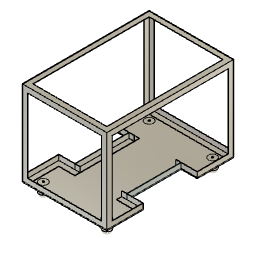
sentry_frame v40 (Autodesk Fusion 360 design; units mm, degrees)
Autodesk Fusion 360 part; units mm, degrees
sketch "1-inch Frame Profile" plane through (0, 0, 0) normal (0, 1, 0) x (1, 0, 0)
  line L0 (-200, -27.4) -> (-200, -2)
  line L1 (-200, -2) -> (-174.6, -2)
  line L2 (-174.6, -2) -> (-174.6, -27.4)
  line L3 (-174.6, -27.4) -> (-200, -27.4)
  line L4 (-174.6, -27.4) -> (-198, -27.4)
  line L5 (-198, -27.4) -> (-198, -4)
  line L6 (-198, -4) -> (-174.6, -4)
  line L7 (-174.6, -4) -> (-174.6, -27.4)
  dimension "d5" = 25.4
  dimension "d6" = 25.4
  dimension "d7" = 23.4
  dimension "d8" = 23.4
  constraint perpendicular L0 L1
  constraint parallel L0 L2
  constraint parallel L1 L3
  constraint vertical L0
  constraint horizontal L4
  constraint vertical L5
  constraint horizontal L6
  constraint vertical L7
  measures "d5" distance of L0.start L2.end
  measures "d6" distance of L1 L3
  measures "d7" distance of L2.end L4.end
  measures "d8" distance of L2.end L6.end
extrude "Extrude3" add sketch "1-inch Frame Profile" along normal blind 600 contours L0 L1 L2 L3 L5 L6 makes body 1
move_body "Move1" bodies 1 to x (1, 0, 0) y (0, 1, 0) z (0, 0, 1) at (0, -300, 0)
copy_body "CopyPasteBodies1" bodies 1 makes body 2
move_body "Move2" bodies 2 to x (-1, 0, 0) y (0, -1, 0) z (0, 0, 1) at (-400, -600, 0)
move_body "Move3" bodies 2 to x (1, 0, 0) y (0, 1, 0) z (0, 0, 1) at (400, 600, 0)
extrude "Extrude5" add sketch "1-inch Frame Profile" along normal blind 400 separate body contours L0 L1 L2 L3 L5 L6 makes body 3
move_body "Move8" bodies 3 to x (0, 1, 0) y (-1, 0, 0) z (0, 0, 1) at (-200, 200, 0)
move_body "Move9" bodies 3 to x (1, 0, 0) y (0, 1, 0) z (0, 0, 1) at (400, -300, 0)
copy_body "CopyPasteBodies4" bodies 3 makes body 4
move_body "Move10" bodies 4 to x (-1, 0, 0) y (0, -1, 0) z (0, 0, 1) at (0, 0, 0)
move_body "Move11" bodies 1 3 4 2 to x (-1, 0, 0) y (0, 1, 0) z (0, 0, -1) at (0, 0, 4)
move_body "Move12" bodies 1 3 4 2 to x (1, 0, 0) y (0, 1, 0) z (0, 0, 1) at (0, 0, 400)
copy_body "CopyPasteBodies5" bodies 3 4 makes body 5 makes body 6
move_body "Move13" bodies 5 6 to x (-1, 0, 0) y (0, 1, 0) z (0, 0, -1) at (0, 0, 778.6)
move_body "Move14" bodies 5 6 to x (1, 0, 0) y (0, 1, 0) z (0, 0, 1) at (0, 0, -375)
extrude "Extrude6" add sketch "1-inch Frame Profile" along normal blind 173 separate body contours L0 L1 L2 L3 L5 L6 makes body 7
move_body "Move15" bodies 7 to x (1, 0, 0) y (0, 1, 0) z (0, 0, 1) at (0, -300, 0)
copy_body "CopyPasteBodies6" bodies 7 makes body 8
move_body "Move16" bodies 8 to x (1, 0, 0) y (0, 1, 0) z (0, 0, 1) at (0, 427, 0)
copy_body "CopyPasteBodies7" bodies 7 8 makes body 9 makes body 10
move_body "Move17" bodies 9 10 to x (-1, 0, 0) y (0, -1, 0) z (0, 0, 1) at (0, 0, 0)
extrude "Extrude7" add sketch "1-inch Frame Profile" along normal blind 101.6 separate body contours L0 L1 L2 L3 L5 L6 makes body 11
move_body "Move18" bodies 11 to x (0, -1, 0) y (1, 0, 0) z (0, 0, 1) at (-200, -327, 0)
copy_body "CopyPasteBodies8" bodies 11 makes body 12
move_body "Move19" bodies 12 to x (-1, 0, 0) y (0, -1, 0) z (0, 0, 1) at (-300, 5.2, 0)
move_body "Move20" bodies 12 to x (1, 0, 0) y (0, 1, 0) z (0, 0, 1) at (1.6, -5.2, 0)
extrude "Extrude8" add sketch "1-inch Frame Profile" along normal blind 254 separate body contours L0 L1 L2 L3 L5 L6 makes body 13
move_body "Move21" bodies 13 to x (1, 0, 0) y (0, 1, 0) z (0, 0, 1) at (76.2, -127, 0)
combine "Combine1" operation add target body 11 tool bodies 13 12
copy_body "CopyPasteBodies9" bodies 11 makes body 14
move_body "Move22" bodies 14 to x (-1, 0, 0) y (0, -1, 0) z (0, 0, 1) at (0, 0, 0)
combine "Combine2" operation add target body 14 tool bodies 9 11 10 7 5 6 8
combine "Combine3" operation add target body 1 tool bodies 4 3 2
extrude "Extrude9" add sketch "1-inch Frame Profile" along normal blind 400 separate body contours L0 L1 L2 L3 L5 L6 makes body 15
move_body "Move23" bodies 15 to x (1, 0, 0) y (0, 0, 1) z (0, -1, 0) at (0, 302, 2)
copy_body "CopyPasteBodies10" bodies 15 makes body 16
move_body "Move24" bodies 16 to x (0, 1, 0) y (-1, 0, 0) z (0, 0, 1) at (99.6, -100, 0)
move_body "Move25" bodies 16 to x (1, 0, 0) y (0, 1, 0) z (0, 0, 1) at (0.4, 0, 0)
copy_body "CopyPasteBodies11" bodies 15 16 makes body 17 makes body 18
move_body "Move26" bodies 17 18 to x (-1, 0, 0) y (0, -1, 0) z (0, 0, 1) at (0, -0.8, 0)
move_body "Move27" bodies 17 18 to x (1, 0, 0) y (0, 1, 0) z (0, 0, 1) at (0, 0.8, 0)
sketch "Sketch7" plane through (0, 0, 0) normal (0, 0, 1) x (1, 0, 0)
  line L0 (-200, 300) -> (200, 300)
  line L1 (200, 300) -> (200, -300)
  line L2 (200, -300) -> (-200, -300)
  line L3 (-200, -300) -> (-200, 300)
  line L4 (123.8, -127) -> (200, -127)
  line L5 (200, -127) -> (200, 127.0447)
  line L6 (200, 127.0447) -> (123.8, 127.0447)
  line L7 (123.8, 127.0447) -> (123.8, -127)
  line L8 (-123.8, -127) -> (-200, -127)
  line L9 (-200, -127) -> (-200, 126.9617)
  line L10 (-200, 126.9617) -> (-123.8, 126.9617)
  line L11 (-123.8, 126.9617) -> (-123.8, -127)
  constraint horizontal L0
  constraint vertical L1
  constraint horizontal L2
  constraint vertical L3
  constraint perpendicular L4 L5
  constraint parallel L4 L6
  constraint parallel L5 L7
  constraint coincident L1 L4.end
  constraint perpendicular L1 L4
  constraint perpendicular L8 L9
  constraint parallel L8 L10
  constraint parallel L9 L11
  constraint coincident L3 L8.end
  constraint perpendicular L3 L8
extrude "Extrude10" add sketch "Sketch7" along normal blind 2 separate body contours L0 L1 L2 L3 L4 L6 L7 L8 L10 L11 makes body 19
sketch "Sketch9" plane through (0, 0, 2) normal (0, 0, 1) x (-1, 0, 0)
  line L0 (200, -126.9617) -> (123.8, -126.9617)
  line L1 (123.8, -126.9617) -> (123.8, 127)
  line L2 (123.8, 127) -> (200, 127)
  line L3 (200, 127) -> (200, 300)
  line L4 (200, 300) -> (-200, 300)
  line L5 (-200, 300) -> (-200, 127)
  line L6 (-200, 127) -> (-123.8, 127)
  line L7 (-123.8, 127) -> (-123.8, -127.0447)
  line L8 (-123.8, -127.0447) -> (-200, -127.0447)
  line L9 (-200, -127.0447) -> (-200, -300)
  line L10 (-200, -300) -> (200, -300)
  line L11 (200, -300) -> (200, -126.9617)
  circle A0 centre (150, 250) radius 4.25
  circle A1 centre (-150, 250) radius 4.25
  circle A2 centre (150, -250) radius 4.25
  circle A3 centre (-150, -250) radius 4.25
  dimension "d30" = 8.5
  dimension "d31" = 8.5
  dimension "d32" = 8.5
  dimension "d33" = 8.5
  measures "d30" diameter of A0
  measures "d31" diameter of A1
  measures "d32" diameter of A2
  measures "d33" diameter of A3
extrude "Extrude12" cut sketch "Sketch9" against normal blind 10 contours A0 | A1 | A2 | A3 bodies 19
combine "Combine4" operation add target body 1 tool bodies 18 17 14 15 16
copy_body "Body->Comp4" bodies 1 removing the originals makes body 20 in component "base_link"
sketch "Sketch14" plane through (123.8, 0, 0) normal (1, 0, 0) x (0, 1, 0)
  line L0 (127, 62) -> (127, 87.4)
  line L1 (127, 87.4) -> (-127, 87.4)
  line L2 (-127, 87.4) -> (-127, 62)
  line L3 (-127, 62) -> (127, 62)
sketch "Sketch17" plane through (-123.8, 0, 0) normal (-1, 0, 0) x (0, -1, 0)
  line L0 (127, 62) -> (127, 87.4)
  line L1 (127, 87.4) -> (-127, 87.4)
  line L2 (-127, 87.4) -> (-127, 62)
  line L3 (-127, 62) -> (127, 62)
sketch "Sketch18" plane through (0, 0, 0) normal (1, 0, 0) x (0, 1, 0)
  circle A0 centre (0, 73) radius 4.4721
copy_body "CutPasteBodies4" bodies 19 body 19 seen with x (1, 0, 0) y (0, 1, 0) z (0, 0, 1) at (0, 0, -60) removing the originals makes body 21 in component "base_link"
move_body "Move3'" bodies 21 to x (1, 0, 0) y (0, 1, 0) z (0, 0, 1) at (0, 0, 60) in component "base_link"
combine "Combine2'" operation add target body 21 tool bodies 20 in component "base_link"
sketch "Sketch30" plane through (0, 0, 60) normal (0, 0, -1) x (1, 0, 0)
  circle A0 centre (150, 250) radius 4.25
  circle A1 centre (150, -250) radius 4.25
  circle A2 centre (-150, 250) radius 4.25
  circle A3 centre (-150, -250) radius 4.25
  line L0 (-123.8, -126.9617) -> (-200, -126.9617)
  line L1 (-200, -126.9617) -> (-200, -300)
  line L2 (-200, -300) -> (200, -300)
  line L3 (200, -300) -> (200, -127.0447)
  line L4 (200, -127.0447) -> (123.8, -127.0447)
  line L5 (123.8, -127.0447) -> (123.8, 127)
  line L6 (123.8, 127) -> (200, 127)
  line L7 (200, 127) -> (200, 300)
  line L8 (200, 300) -> (-200, 300)
  line L9 (-200, 300) -> (-200, 127)
  line L10 (-200, 127) -> (-123.8, 127)
  line L11 (-123.8, 127) -> (-123.8, -126.9617)
  circle A4 centre (-150, 250) radius 20
  dimension "d284" = 40
  constraint concentric A2 A4
  measures "d284" diameter of A4
extrude "Extrude1" add sketch "Sketch30" along normal blind 60 contours A2 | A4 sketch seen with x (1, 0, 0) y (0, 1, 0) z (0, 0, 1) at (0, 0, -60) bodies 21 in component "base_link"
fillet "Fillet1" radius 20 1 edges at (-168.6465, -242.7677, -60) on bodies 21 in component "base_link"
sketch "Sketch31" plane through (0, 0, 60) normal (0, 0, -1) x (1, 0, 0)
  circle A0 centre (-150, 250) radius 20
  circle A1 centre (150, 250) radius 4.25
  circle A2 centre (150, -250) radius 4.25
  circle A3 centre (-150, -250) radius 4.25
  line L0 (-123.8, -126.9617) -> (-200, -126.9617)
  line L1 (-200, -126.9617) -> (-200, -300)
  line L2 (-200, -300) -> (200, -300)
  line L3 (200, -300) -> (200, -127.0447)
  line L4 (200, -127.0447) -> (123.8, -127.0447)
  line L5 (123.8, -127.0447) -> (123.8, 127)
  line L6 (123.8, 127) -> (200, 127)
  line L7 (200, 127) -> (200, 300)
  line L8 (200, 300) -> (-200, 300)
  line L9 (-200, 300) -> (-200, 127)
  line L10 (-200, 127) -> (-123.8, 127)
  line L11 (-123.8, 127) -> (-123.8, -126.9617)
  circle A4 centre (150, 250) radius 20
  dimension "d289" = 40
  constraint concentric A1 A4
  measures "d289" diameter of A4
extrude "Extrude2" add sketch "Sketch31" along normal blind 60 contours A1 | A4 sketch seen with x (1, 0, 0) y (0, 1, 0) z (0, 0, 1) at (0, 0, -60) bodies 21 in component "base_link"
fillet "Fillet2" radius 20 1 faces at (156.1685, -243.352, -60) on bodies 21 in component "base_link"
sketch "Sketch32" plane through (0, 0, 60) normal (0, 0, -1) x (1, 0, 0)
  circle A0 centre (150, 250) radius 20
  circle A1 centre (-150, 250) radius 20
  circle A2 centre (150, -250) radius 4.25
  circle A3 centre (-150, -250) radius 4.25
  line L0 (-123.8, -126.9617) -> (-200, -126.9617)
  line L1 (-200, -126.9617) -> (-200, -300)
  line L2 (-200, -300) -> (200, -300)
  line L3 (200, -300) -> (200, -127.0447)
  line L4 (200, -127.0447) -> (123.8, -127.0447)
  line L5 (123.8, -127.0447) -> (123.8, 127)
  line L6 (123.8, 127) -> (200, 127)
  line L7 (200, 127) -> (200, 300)
  line L8 (200, 300) -> (-200, 300)
  line L9 (-200, 300) -> (-200, 127)
  line L10 (-200, 127) -> (-123.8, 127)
  line L11 (-123.8, 127) -> (-123.8, -126.9617)
  circle A4 centre (-150, -250) radius 20
  dimension "d294" = 40
  constraint concentric A3 A4
  measures "d294" diameter of A4
extrude "Extrude3'" add sketch "Sketch32" along normal blind 60 contours A3 | A4 sketch seen with x (1, 0, 0) y (0, 1, 0) z (0, 0, 1) at (0, 0, -60) bodies 21 in component "base_link"
fillet "Fillet3" radius 20 1 faces at (-144.9812, 239.0673, -60) on bodies 21 in component "base_link"
sketch "Sketch33" plane through (0, 0, 60) normal (0, 0, -1) x (1, 0, 0)
  circle A0 centre (-150, -250) radius 20
  circle A1 centre (150, 250) radius 20
  circle A2 centre (-150, 250) radius 20
  circle A3 centre (150, -250) radius 4.25
  line L0 (-123.8, -126.9617) -> (-200, -126.9617)
  line L1 (-200, -126.9617) -> (-200, -300)
  line L2 (-200, -300) -> (200, -300)
  line L3 (200, -300) -> (200, -127.0447)
  line L4 (200, -127.0447) -> (123.8, -127.0447)
  line L5 (123.8, -127.0447) -> (123.8, 127)
  line L6 (123.8, 127) -> (200, 127)
  line L7 (200, 127) -> (200, 300)
  line L8 (200, 300) -> (-200, 300)
  line L9 (-200, 300) -> (-200, 127)
  line L10 (-200, 127) -> (-123.8, 127)
  line L11 (-123.8, 127) -> (-123.8, -126.9617)
  circle A4 centre (150, -250) radius 20
  dimension "d299" = 40
  constraint concentric A3 A4
  measures "d299" diameter of A4
extrude "Extrude4" add sketch "Sketch33" along normal blind 60 contours A3 | A4 sketch seen with x (1, 0, 0) y (0, 1, 0) z (0, 0, 1) at (0, 0, -60) bodies 21 in component "base_link"
fillet "Fillet4" radius 20 1 faces at (155.0188, 239.0673, -60) on bodies 21 in component "base_link"
component "base_link" placed x (1, 0, 0) y (0, 1, 0) z (0, 0, 1) at (0, 0, 60)
named bodies: "Frame", "Frame_longEdge_2", "Frame_shortEdge_1", "Frame_shortEdge_2", "Frame_shortEdge_1 (1)", "Frame_shortEdge_2 (1)", "Frame_wheelEdge_1", "Frame_wheelEdge_1 (1)", "Frame_wheelEdge_1 (1) (1)", "Frame_wheelEdge_1 (1) (1) (1)", "Frame_wheelWell", "Frame_wheelWell (1)", "Frame_wheelWell (2)", "Frame_stand", "Frame_stand (1)", "Frame_stand (1) (1)", "Frame_stand (1) (1) (1)", "Base_Plate", "frame"
